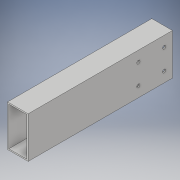
# Autodesk Inventor part: 1x2 Placeholder
Saved by Autodesk Inventor 2018 (Build 220112000, 112)
## iProperties
Created: 2020-01-28
Part Number: 1x2 Placeholder
Material: Generic
Document SubType Name: Modeling
Designer: maste
Density: 1 g/cm^3
Appearance: Default
Author: maste
Autodesk Inventor part; units mm, degrees
ref_plane "YZ Plane" through (0, 0, 0) normal (1, 0, 0) x (0, 1, 0)
ref_plane "XZ Plane" through (0, 0, 0) normal (0, 1, 0) x (-1, 0, 0)
ref_plane "XY Plane" through (0, 0, 0) normal (0, 0, 1) x (1, 0, 0)
sketch "Sketch1" plane through (0, 0, 0) normal (0, 0, 1) x (1, 0, 0)
  line L0 (0, 0) -> (25.4, 0)
  line L1 (25.4, 0) -> (25.4, 50.8)
  line L2 (25.4, 50.8) -> (0, 50.8)
  line L3 (0, 50.8) -> (0, 0)
  line L4 (23.8125, 49.2125) -> (23.8125, 1.5875)
  line L5 (23.8125, 1.5875) -> (1.5875, 1.5875)
  line L6 (1.5875, 1.5875) -> (1.5875, 49.2125)
  line L7 (1.5875, 49.2125) -> (23.8125, 49.2125)
  dimension "d0" = 25.4
  dimension "d1" = 50.8
  dimension "d2" = 1.5875
  constraints: 16 end point, 4 parallel, 2 perpendicular, 1 horizontal, 3 other
  measures "d0" distance of L2.end L1.end
  measures "d1" distance of L1.end L0.end
  measures "d2" distance between parallel lines of L1 L4
extrude "Extrusion1" add sketch "Sketch1" along normal blind 177.8
sketch "Sketch2" plane through (25.4, 0, 0) normal (1, 0, 0) x (0, 0, -1)
  line L0 (0, 1.5875) -> (0, 49.2125) construction
  line L1 (0, 25.4) -> (0, 38.1) construction
  line L2 (0, 38.1) -> (-10.2108, 38.1) construction
  line L3 (-10.2108, 38.1) -> (-10.2108, 12.7) construction
  line L4 (-10.2108, 12.7) -> (-41.9608, 12.7) construction
  line L5 (-41.9608, 12.7) -> (-41.9608, 38.1) construction
  circle A0 centre (-10.2108, 38.1) radius 2.0193
  circle A1 centre (-10.2108, 12.7) radius 2.0193
  circle A2 centre (-41.9608, 12.7) radius 2.0193
  circle A3 centre (-41.9608, 38.1) radius 2.0193
  point P0 (0, 0)
  dimension "d5" = 12.7
  dimension "d6" = 10.2108
  dimension "d7" = 25.4
  dimension "d9" = 31.75
  dimension "d10" = 4.0386
  constraints: 10 end point, 4 centre point, 4 coincident, 3 perpendicular, 1 horizontal, 1 midpoint, 1 point on line
  measures "d5" distance of L1.start L1.end
  measures "d6" distance of L1.end L2.end
  measures "d7" distance of L2.end L3.end
  measures "d9" distance of L3.end L4.end
  measures "d10" diameter of A0
extrude "Extrusion2" cut sketch "Sketch2" against normal blind 177.8
body "Solid1"
